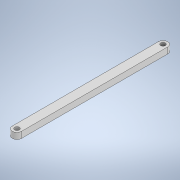
# Autodesk Inventor part: link-2
Saved by Autodesk Inventor 2020 (Build 240168000, 168)
## iProperties
Created: 2020-11-06
Part Number: link-2
Material: Generic
Document SubType Name: Modeling
Designer: alnwlsn
Density: 1 g/cm^3
Appearance: Default
Author: alnwlsn
Autodesk Inventor part; units mm, degrees
ref_plane "YZ Plane" through (0, 0, 0) normal (1, 0, 0) x (0, 1, 0)
ref_plane "XZ Plane" through (0, 0, 0) normal (0, 1, 0) x (-1, 0, 0)
ref_plane "XY Plane" through (0, 0, 0) normal (0, 0, 1) x (1, 0, 0)
sketch "Sketch1" plane through (0, 0, 0) normal (0, 1, 0) x (-1, 0, 0)
  line L0 (0, 0) -> (0, -47.7) construction
  line L1 (1.5, 0) -> (1.5, -47.7)
  line L2 (-1.5, -47.7) -> (-1.5, 0)
  arc A0 (1.5, 0) -> (-1.5, 0) centre (0, 0) ccw
  arc A1 (-1.5, -47.7) -> (1.5, -47.7) centre (0, -47.7) ccw
  circle A2 centre (0, 0) radius 0.75
  circle A3 centre (0, -47.7) radius 0.75
  point P0 (0, -23.85)
  dimension "d0" = 3
  dimension "d1" = 1.5
  dimension "d2" = 47.7
  constraints: 8 end point, 4 centre point, 4 point on circle, 4 tangent, 2 coincident, 1 equal radius, 1 midpoint, 1 parallel, 1 vertical
  measures "d0" distance between parallel lines of L2 L1
  measures "d1" diameter of A2
  measures "d2" distance of L0.start L0.end
extrude "Extrusion1" add sketch "Sketch1" along normal blind 2
body "Solid1"
